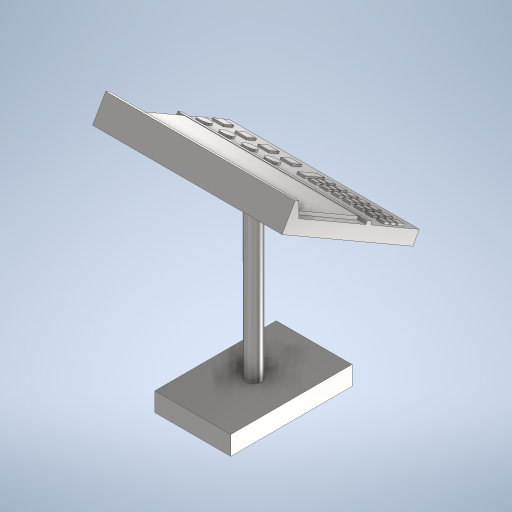
# Autodesk Inventor part: ctrl_panel
Saved by Autodesk Inventor 2023 (Build 270158000, 158)
## iProperties
Created: 2023-11-22
Part Number: ctrl_panel
Material: Generic
Document SubType Name: Modeling
Designer: Beatrice
Density: 1 g/cm^3
Appearance: Semi-Polished
Author: Beatrice
Autodesk Inventor part; units mm, degrees
ref_plane "YZ Plane" through (0, 0, 0) normal (1, 0, 0) x (0, 1, 0)
ref_plane "XZ Plane" through (0, 0, 0) normal (0, 1, 0) x (-1, 0, 0)
ref_plane "XY Plane" through (0, 0, 0) normal (0, 0, 1) x (1, 0, 0)
sketch "Sketch1" plane through (0, 0, 0) normal (1, 0, 0) x (0, 1, 0)
  line L0 (-2, 0) -> (2, 0)
  line L1 (2, 0) -> (2, 50)
  line L2 (2, 50) -> (-2, 50)
  line L3 (-2, 50) -> (-2, 0)
  line L4 (-16, 0) -> (16, 0)
  line L5 (16, 0) -> (16, 5)
  line L6 (16, 5) -> (-16, 5)
  line L7 (-16, 5) -> (-16, 0)
  line L8 (-2, 50) -> (17.0526, 39)
  line L9 (-2, 50) -> (20, 50) construction
  line L10 (17.0526, 39) -> (20.5167, 45)
  line L11 (20.5167, 45) -> (-14, 64.9282)
  line L12 (-14, 64.9282) -> (-17.4641, 58.9282)
  line L13 (-17.4641, 58.9282) -> (-1.5322, 49.7299)
  line L14 (-13, 64.3509) -> (-13, 60.3509)
  line L15 (-13, 64.3509) -> (-9, 64.3509) construction
  line L16 (-13, 60.3509) -> (18.7846, 42)
  line L17 (0, 0) -> (0, 60.3509)
  point P0 (0, 48.8453)
  dimension "d0" = 2
  dimension "d1" = 50
  dimension "d2" = 30
  dimension "d3" = 90
  constraints: 36 end point, 5 perpendicular, 4 horizontal, 4 parallel, 3 midpoint, 3 point on line, 2 equal length, 1 coincident, 1 vertical
  measures "d0" distance from line of point (0, 0) L3
  measures "d1" distance of L0.end L1.end
  measures "d2" angle of L8 L9
  measures "d3" angle of L14 L15
extrude "Extrusion1" add sketch "Sketch1" along normal mid plane 50 contours L13 L12 L11 L14 L16 L17 L2 | L2 L17 L8 | L17 L2 L1 L8 | L17 L16 L10 L8 L1 L2
sketch "Sketch2" plane through (-25, -13, 60.3509) normal (0, 0.5, 0.8660254) x (1, 0, 0)
  line L0 (0, 0) -> (50, 0) projected
  line L1 (50, 36.7017) -> (50, 0) projected
  line L2 (0, 36.7017) -> (50, 36.7017) projected
  line L3 (0, 0) -> (0, 36.7017) projected
  line L4 (50, -3.1547) -> (50, 36.7017) projected
  line L5 (0, 34) -> (50, 34)
  line L6 (50, 34) -> (50, 22)
  line L7 (50, 22) -> (0, 22)
  line L8 (0, 22) -> (0, 34)
  line L9 (1, 33) -> (4, 33)
  line L10 (4, 33) -> (4, 30)
  line L11 (4, 30) -> (1, 30)
  line L12 (1, 30) -> (1, 33)
  line L13 (0, 25.8225) -> (50, 25.8225)
  line L14 (2.5, 22) -> (2.5, 34)
  circle A0 centre (2.5, 25.8225) radius 1.7107
  line L15 (26, 33) -> (49, 33)
  line L16 (49, 33) -> (49, 27)
  line L17 (49, 27) -> (26, 27)
  line L18 (26, 27) -> (26, 33)
  line L19 (26, 33) -> (28, 33)
  line L20 (28, 33) -> (28, 27)
  line L21 (28, 27) -> (26, 27)
  line L22 (26, 27) -> (26, 33)
  line L23 (29, 33) -> (31, 33)
  line L24 (31, 33) -> (31, 27)
  line L25 (31, 27) -> (29, 27)
  line L26 (29, 27) -> (29, 33)
  line L27 (32, 33) -> (34, 33)
  line L28 (34, 33) -> (34, 27)
  line L29 (34, 27) -> (32, 27)
  line L30 (32, 27) -> (32, 33)
  line L31 (35, 33) -> (37, 33)
  line L32 (37, 33) -> (37, 27)
  line L33 (37, 27) -> (35, 27)
  line L34 (35, 27) -> (35, 33)
  line L35 (38, 33) -> (40, 33)
  line L36 (40, 33) -> (40, 27)
  line L37 (40, 27) -> (38, 27)
  line L38 (38, 27) -> (38, 33)
  line L39 (41, 33) -> (43, 33)
  line L40 (43, 33) -> (43, 27)
  line L41 (43, 27) -> (41, 27)
  line L42 (41, 27) -> (41, 33)
  line L43 (44, 33) -> (46, 33)
  line L44 (46, 33) -> (46, 27)
  line L45 (46, 27) -> (44, 27)
  line L46 (44, 27) -> (44, 33)
  line L47 (47, 33) -> (49, 33)
  line L48 (49, 33) -> (49, 27)
  line L49 (49, 27) -> (47, 27)
  line L50 (47, 27) -> (47, 33)
  line L51 (26, 31) -> (49, 31)
  line L52 (26, 28.5023) -> (49, 28.5023)
  line L53 (26, 30.5291) -> (49, 30.5291)
  line L54 (26, 29) -> (49, 29)
  line L55 (7, 30) -> (7, 33)
  line L56 (7, 33) -> (10, 33)
  line L57 (10, 33) -> (10, 30)
  line L58 (10, 30) -> (7, 30)
  circle A1 centre (8.5, 25.8225) radius 1.7107
  line L59 (13, 30) -> (13, 33)
  line L60 (13, 33) -> (16, 33)
  line L61 (16, 33) -> (16, 30)
  line L62 (16, 30) -> (13, 30)
  circle A2 centre (14.5, 25.8225) radius 1.7107
  line L63 (19, 30) -> (19, 33)
  line L64 (19, 33) -> (22, 33)
  line L65 (22, 33) -> (22, 30)
  line L66 (22, 30) -> (19, 30)
  circle A3 centre (20.5, 25.8225) radius 1.7107
  point P0 (25, 41.4338)
  point P1 (31, 28.5023)
  point P2 (29, 28.5023)
  point P3 (29, 29)
  point P4 (31, 29)
  point P5 (31, 30.5291)
  point P6 (29, 30.5291)
  point P7 (32, 29)
  point P8 (34, 29)
  point P9 (34, 30.5291)
  point P10 (32, 30.5291)
  point P11 (34, 28.5023)
  point P12 (32, 28.5023)
  point P13 (37, 28.5023)
  point P14 (35, 28.5023)
  point P15 (35, 29)
  point P16 (37, 29)
  point P17 (37, 30.5291)
  point P18 (35, 30.5291)
  point P19 (38, 29)
  point P20 (40, 29)
  point P21 (40, 30.5291)
  point P22 (38, 30.5291)
  point P23 (40, 28.5023)
  point P24 (38, 28.5023)
  point P25 (43, 28.5023)
  point P26 (41, 28.5023)
  point P27 (41, 29)
  point P28 (43, 29)
  point P29 (43, 30.5291)
  point P30 (41, 30.5291)
  point P31 (44, 29)
  point P32 (46, 29)
  point P33 (46, 30.5291)
  point P34 (44, 30.5291)
  point P35 (46, 28.5023)
  point P36 (44, 28.5023)
  point P37 (47, 28.5023)
  point P38 (47, 29)
  point P39 (49, 29)
  point P40 (47, 30.5291)
  point P41 (47, 31)
  point P42 (49, 31)
  point P43 (44, 31)
  point P44 (46, 31)
  point P45 (46, 33)
  point P46 (41, 31)
  point P47 (43, 31)
  point P48 (43, 33)
  point P49 (38, 31)
  point P50 (40, 31)
  point P51 (40, 33)
  point P52 (35, 31)
  point P53 (37, 31)
  point P54 (37, 33)
  point P55 (32, 31)
  point P56 (34, 31)
  point P57 (34, 33)
  point P58 (29, 31)
  point P59 (31, 31)
  point P60 (31, 33)
  point P61 (28, 33)
  dimension "d6" = 3
  dimension "d13" = 6
  constraints: 120 end point, 21 parallel, 16 perpendicular, 15 point on line, 11 horizontal, 4 centre point, 1 vertical, 50 other
  measures "d6" distance between parallel lines of L11 L9
  measures "d13" distance of L11.end L55.start
extrude "Extrusion2" add sketch "Sketch2" along normal blind 0.5 and the other way blind 0.15 contours A0 L14 L13 | L13 L14 A0 | L14 L13 A0 | A3 L13 | L13 A3 | L14 A0 L13 | L14 L11 L12 L9 | L9 L10 L11 L14 | A1 L13 | L13 A1 | A2 L13 | L13 A2 | L15 L20 L51 L18 | L51 L20 L53 L18 | L15 L24 L51 L26 | L53 L20 L54 L18 | L54 L20 L52 L18 | L15 L28 L51 L30 | L53 L24 L54 L26 | L52 L20 L17 L18 | L15 L32 L51 L34 | L53 L28 L54 L30 | L52 L24 L17 L26 | L15 L36 L51 L38 | L53 L32 L54 L34 | L52 L28 L17 L30 | L15 L40 L51 L42 | L53 L36 L54 L38 | L52 L32 L17 L34 | L15 L44 L51 L46 | L53 L40 L54 L42 | L52 L36 L17 L38 | L15 L16 L51 L50 | L53 L44 L54 L46 | L52 L40 L17 L42 | L53 L16 L54 L50 | L52 L44 L17 L46 | L52 L16 L17 L50 | L55 L56 L57 L58 | L59 L60 L61 L62 | L63 L64 L65 L66
sketch "Sketch3" plane through (-25, -13, 60.3509) normal (0, 0.5, 0.8660254) x (1, 0, 0)
  line L0 (48, 2) -> (2, 2)
  line L1 (2, 2) -> (2, 20)
  line L2 (2, 20) -> (48, 20)
  line L3 (48, 20) -> (48, 2)
  line L4 (50, -3.1547) -> (50, 36.7017) projected
  line L5 (0, 36.7017) -> (0, -3.1547) projected
  line L6 (50, 20.3737) -> (0, 20.3737)
  line L7 (0, 20.3737) -> (0, 21.5188)
  line L8 (0, 21.5188) -> (50, 21.5188)
  line L9 (50, 21.5188) -> (50, 20.3737)
  point P0 (25, 41.4338)
  point P1 (50, 21.5188)
  constraints: 16 end point, 4 parallel, 2 horizontal, 2 perpendicular, 2 point on line
extrude "Extrusion3" add sketch "Sketch3" along normal blind 0.8
revolve "Revolution1" add sketch "Sketch1" angle 360 about axis through (0, 0, 0) along (0, 0, 1) contours L3 L6 L17 L0 | L3 L8 L17 L6
extrude "Extrusion4" add sketch "Sketch1" along normal mid plane 20 contours L3 L6 L17 L0 | L4 L7 L6 L3 | L17 L6 L1 L0 | L1 L6 L5 L4
fillet "Fillet1" radius 1 1 edges at (0, 5.6358, 49.5915)
body "Solid1"
